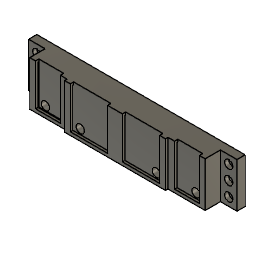
charging_plate (Autodesk Fusion 360 design; units mm, degrees)
part number: 2026-05-24-20-13-33-202
Autodesk Fusion 360 part; units mm, degrees
sketch "Sketch1" plane through (0, 0, 0) normal (0, 1, 0) x (1, 0, 0)
  line L0 (0, 0) -> (252, 0)
  line L1 (252, 0) -> (252, -54.2)
  line L2 (252, -54.2) -> (0, -54.2)
  line L3 (0, -54.2) -> (0, 0)
  dimension "d1" = 252
  dimension "d2" = 54.2
  constraint horizontal L0
  constraint vertical L1
  constraint horizontal L2
  constraint vertical L3
  constraint coincident L0.start L3.end
  measures "d1" distance of L0.start L0.end
  measures "d2" distance of L0.start L2.end
extrude "Extrude1" add sketch "Sketch1" along normal blind 10
sketch "Sketch2" plane through (0, 0, 0) normal (0, -1, 0) x (1, 0, 0)
  line L0 (252, 54.2) -> (0, 54.2)
  line L1 (0, 54.2) -> (0, 0)
  line L2 (0, 0) -> (252, 0)
  line L3 (252, 0) -> (252, 54.2)
  line L4 (20, 54.2) -> (232, 54.2)
  line L5 (232, 54.2) -> (232, 0)
  line L6 (232, 0) -> (20, 0)
  line L7 (20, 0) -> (20, 54.2)
  dimension "d5" = 20
  dimension "d6" = 20
  constraint horizontal L4
  constraint vertical L5
  constraint horizontal L6
  constraint vertical L7
  constraint coincident L2 L5.end
  constraint coincident L0 L4.start
  measures "d5" distance of L1.end L6.end
  measures "d6" distance of L2.end L5.end
extrude "Extrude2" add sketch "Sketch2" along normal blind 18.5 contours L0 L2 L4 L5 L6 L7
sketch "Sketch3" plane through (0, -18.5, 0) normal (0, -1, 0) x (1, 0, 0)
  line L0 (20, 0) -> (232, 0)
  line L1 (232, 0) -> (232, 54.2)
  line L2 (232, 54.2) -> (20, 54.2)
  line L3 (20, 54.2) -> (20, 0)
  line L4 (65, 54.2) -> (187, 54.2)
  line L5 (187, 54.2) -> (187, 0)
  line L6 (187, 0) -> (65, 0)
  line L7 (65, 0) -> (65, 54.2)
  dimension "d9" = 45
  dimension "d10" = 45
  constraint horizontal L4
  constraint vertical L5
  constraint horizontal L6
  constraint vertical L7
  constraint coincident L0 L5.end
  constraint coincident L2 L4.start
  measures "d9" distance of L0.start L6.end
  measures "d10" distance of L0.end L5.end
extrude "Extrude3" add sketch "Sketch3" along normal blind 3 contours L0 L2 L4 L5 L6 L7
sketch "Sketch4" plane through (0, -18.5, 0) normal (0, -1, 0) x (1, 0, 0)
  line L0 (65, 0) -> (65, 54.2)
  line L1 (65, 54.2) -> (20, 54.2)
  line L2 (20, 54.2) -> (20, 0)
  line L3 (20, 0) -> (65, 0)
  line L4 (27, 54.2) -> (57, 54.2)
  line L5 (57, 54.2) -> (57, 4)
  line L6 (57, 4) -> (27, 4)
  line L7 (27, 4) -> (27, 54.2)
  line L8 (195, 54.2) -> (225, 54.2)
  line L9 (225, 54.2) -> (225, 4)
  line L10 (225, 4) -> (195, 4)
  line L11 (195, 4) -> (195, 54.2)
  line L12 (232, 0) -> (252, 0)
  point P0 (232, 54.2)
  dimension "d13" = 7
  dimension "d14" = 30
  dimension "d15" = 4
  dimension "d16" = 7
  dimension "d17" = 30
  dimension "d18" = 4
  constraint horizontal L4
  constraint vertical L5
  constraint horizontal L6
  constraint vertical L7
  constraint coincident L1 L4.start
  constraint horizontal L8
  constraint vertical L9
  constraint horizontal L10
  constraint vertical L11
  measures "d13" distance of L1.end L4.start
  measures "d14" distance of L4.start L4.end
  measures "d15" distance of L3 L5.end
  measures "d16" distance of L8.end P0
  measures "d17" distance of L8.start L8.end
  measures "d18" distance of L9.end L12
extrude "Extrude4" cut sketch "Sketch4" against normal blind 4 contours L1 L4 L5 L6 L7 | L8 L9 L10 L11
sketch "Sketch5" plane through (0, 0, 4) normal (0, 0, 1) x (-1, 0, 0)
  line L0 (-27, 18.5) -> (-57, 18.5)
  line L1 (-57, 18.5) -> (-57, 14.5)
  line L2 (-57, 14.5) -> (-27, 14.5)
  line L3 (-27, 14.5) -> (-27, 18.5)
  line L4 (-24, 14.5285) -> (-59.9999, 14.5285)
  line L5 (-59.9999, 14.5285) -> (-59.9999, 15.5285)
  line L6 (-59.9999, 15.5285) -> (-24, 15.5285)
  line L7 (-24, 15.5285) -> (-24, 14.5285)
  line L8 (-192, 14.5) -> (-228, 14.5)
  line L9 (-228, 14.5) -> (-228, 15.5)
  line L10 (-228, 15.5) -> (-192, 15.5)
  line L11 (-192, 15.5) -> (-192, 14.5)
  line L12 (-195, 18.5) -> (-187, 18.5)
  point P0 (-195, 14.5)
  point P1 (-225, 14.5)
  dimension "d22" = 3
  dimension "d23" = 1
  dimension "d26" = 1
  dimension "d56" = 3
  dimension "d57" = 3
  dimension "d58" = 3
  dimension "d59" = 3
  constraint horizontal L4
  constraint vertical L5
  constraint horizontal L6
  constraint vertical L7
  constraint horizontal L8
  constraint vertical L9
  constraint horizontal L10
  constraint vertical L11
  measures "d22" distance of L1.end L4.end
  measures "d23" distance of L4.start L6.end
  measures "d26" distance of L8.end L9.end
  measures "d56" horizontal distance of L2.end L4.start
  measures "d57" distance of L8.start P0
  measures "d58" distance of L8.end P1
  measures "d59" distance of L10.end L12
extrude "Extrude5" cut sketch "Sketch5" along normal blind 47.2 and the other way blind 3 contours L3 L4 L6 L7 | L1 L3 L4 L6 | L1 L4 L5 L6 | L8 L9 L10 L11
sketch "Sketch6" plane through (0, -21.5, 0) normal (0, -1, 0) x (1, 0, 0)
  line L0 (65, 0) -> (187, 0)
  line L1 (187, 0) -> (187, 54.2)
  line L2 (187, 54.2) -> (65, 54.2)
  line L3 (65, 54.2) -> (65, 0)
  line L4 (72, 54.2) -> (117, 54.2)
  line L5 (117, 54.2) -> (117, 4)
  line L6 (117, 4) -> (72, 4)
  line L7 (72, 4) -> (72, 54.2)
  line L8 (180, 54.2) -> (135, 54.2)
  line L9 (135, 54.2) -> (135, 4)
  line L10 (135, 4) -> (180, 4)
  line L11 (180, 4) -> (180, 54.2)
  dimension "d31" = 7
  dimension "d32" = 45
  dimension "d33" = 4
  dimension "d34" = 7
  dimension "d35" = 45
  dimension "d36" = 4
  constraint horizontal L4
  constraint vertical L5
  constraint horizontal L6
  constraint vertical L7
  constraint coincident L2 L4.start
  constraint horizontal L8
  constraint vertical L9
  constraint horizontal L10
  constraint vertical L11
  constraint coincident L2 L8.start
  measures "d31" distance of L2.end L4.start
  measures "d32" distance of L4.start L4.end
  measures "d33" distance of L0 L6.end
  measures "d34" distance of L1.end L8.start
  measures "d35" distance of L8.start L8.end
  measures "d36" distance of L0 L9.end
extrude "Extrude6" cut sketch "Sketch6" against normal blind 4 contours L2 L4 L5 L6 L7 | L2 L8 L9 L10 L11
sketch "Sketch7" plane through (0, 0, 4) normal (0, 0, 1) x (-1, 0, 0)
  line L0 (-72, 21.5) -> (-117, 21.5)
  line L1 (-117, 17.5) -> (-72, 17.5)
  line L2 (-72, 17.5) -> (-72, 21.5)
  line L3 (-69, 17.5) -> (-120, 17.5)
  line L4 (-120, 17.5) -> (-120, 18.5)
  line L5 (-120, 18.5) -> (-69, 18.5)
  line L6 (-69, 18.5) -> (-69, 17.5)
  line L7 (-132, 17.5) -> (-183, 17.5)
  line L8 (-183, 17.5) -> (-183, 18.5)
  line L9 (-183, 18.5) -> (-132, 18.5)
  line L10 (-132, 18.5) -> (-132, 17.5)
  line L11 (-117, 21.5) -> (-117, 17.5)
  line L12 (-187, 21.5) -> (-180, 21.5)
  line L13 (-72, 21.5) -> (-65, 21.5)
  point P0 (-180, 17.5)
  point P1 (-135, 17.5)
  dimension "d41" = 1
  dimension "d45" = 1
  dimension "d60" = 3
  dimension "d61" = 3
  dimension "d62" = 3
  dimension "d63" = 3
  dimension "d64" = 3
  dimension "d65" = 3
  constraint horizontal L3
  constraint vertical L4
  constraint horizontal L5
  constraint vertical L6
  constraint horizontal L7
  constraint vertical L8
  constraint horizontal L9
  constraint vertical L10
  measures "d41" distance of L3.start L5.end
  measures "d45" distance of L7.end L8.end
  measures "d60" distance of L8.end L12
  measures "d61" distance of L7.end P0
  measures "d62" distance of L7.start P1
  measures "d63" distance of L5.end L13
  measures "d64" distance of L1.start L3.end
  measures "d65" distance of L1.end L3.start
extrude "Extrude7" cut sketch "Sketch7" along normal blind 47.2 and the other way blind 3 contours L2 L3 L5 L6 | L1 L2 L3 L5 L11 | L3 L4 L5 L11 | L7 L8 L9 L10
sketch "Sketch8" plane through (0, 10, 0) normal (0, 1, 0) x (-1, 0, 0)
  line L0 (0, 54.2) -> (-252, 54.2)
  line L1 (-252, 54.2) -> (-252, 0)
  line L2 (-252, 0) -> (0, 0)
  line L3 (0, 0) -> (0, 54.2)
  line L4 (-225, 44.2) -> (-27, 44.2)
  line L5 (-27, 44.2) -> (-27, 10)
  line L6 (-27, 10) -> (-225, 10)
  line L7 (-225, 10) -> (-225, 44.2)
  dimension "d50" = 27
  dimension "d51" = 27
  dimension "d52" = 10
  dimension "d53" = 10
  constraint horizontal L4
  constraint vertical L5
  constraint horizontal L6
  constraint vertical L7
  measures "d50" distance of L1 L7
  measures "d51" distance of L3 L5
  measures "d52" distance of L0 L4
  measures "d53" distance of L2 L6
extrude "Extrude8" cut sketch "Sketch8" against normal blind 20 contours L4 L5 L6 L7
sketch "Sketch9" plane through (0, -10, 0) normal (0, 1, 0) x (-1, 0, 0)
  line L0 (-225, 10) -> (-27, 10)
  line L1 (-27, 10) -> (-27, 44.2)
  line L2 (-27, 44.2) -> (-225, 44.2)
  line L3 (-225, 44.2) -> (-225, 10)
  circle A0 centre (-217, 9.2) radius 5
  circle A1 centre (-172, 9.2) radius 5
  circle A2 centre (-80, 9.2) radius 5
  circle A3 centre (-35, 9.2) radius 5
  line L4 (-252, 54.2) -> (-252, 0)
  line L5 (0, 54.2) -> (0, 0)
  line L6 (0, 54.2) -> (-252, 54.2)
  dimension "d66" = 10
  dimension "d67" = 80
  dimension "d68" = 35
  dimension "d69" = 35
  dimension "d70" = 80
  dimension "d71" = 45
  dimension "d72" = 45
  dimension "d73" = 45
  dimension "d74" = 45
  constraint equal A0 A1
  constraint equal A0 A2
  constraint equal A0 A3
  measures "d66" diameter of A0
  measures "d67" distance of A1.centre L4
  measures "d68" distance of A0.centre L4
  measures "d69" distance of A3.centre L5
  measures "d70" distance of A2.centre L5
  measures "d71" distance of A0.centre L6
  measures "d72" distance of A1.centre L6
  measures "d73" distance of A2.centre L6
  measures "d74" distance of A3.centre L6
extrude "Extrude9" cut sketch "Sketch9" along normal up to surface (-7.5 mm away) and the other way up to surface (-20 mm away) contours L0 A0 | L0 A0 | L0 A1 | L0 A1 | L0 A3 | L0 A3 | L0 A2 | L0 A2
sketch "Sketch10" plane through (0, 0, 0) normal (0, -1, 0) x (1, 0, 0)
  line L0 (20, 0) -> (20, 54.2)
  line L1 (20, 54.2) -> (0, 54.2)
  line L2 (0, 54.2) -> (0, 0)
  line L3 (0, 0) -> (20, 0)
  circle A0 centre (10, 27.1) radius 5
  circle A1 centre (10, 10) radius 5
  circle A2 centre (10, 44.2) radius 5
  circle A3 centre (242, 27.1) radius 5
  circle A4 centre (242, 44.2) radius 5
  circle A5 centre (242, 10) radius 5
  line L4 (252, 0) -> (252, 54.2)
  line L5 (232, 0) -> (252, 0)
  line L6 (252, 54.2) -> (232, 54.2)
  dimension "d77" = 10
  dimension "d78" = 10
  dimension "d79" = 27.1
  dimension "d80" = 10
  dimension "d81" = 10
  dimension "d82" = 10
  dimension "d83" = 10
  dimension "d84" = 10
  dimension "d85" = 10
  dimension "d86" = 10
  dimension "d87" = 27.1
  dimension "d88" = 10
  dimension "d89" = 10
  constraint equal A0 A2
  constraint equal A0 A1
  constraint equal A0 A5
  constraint equal A0 A4
  constraint equal A0 A3
  measures "d77" diameter of A0
  measures "d78" distance of L2 A0.centre
  measures "d79" distance of L3 A0.centre
  measures "d80" distance of L2 A2.centre
  measures "d81" distance of L2 A1.centre
  measures "d82" distance of L1 A2.centre
  measures "d83" distance of L3 A1.centre
  measures "d84" distance of A3.centre L4
  measures "d85" distance of A4.centre L4
  measures "d86" distance of A5.centre L4
  measures "d87" distance of A3.centre L5
  measures "d88" distance of A4.centre L6
  measures "d89" distance of A5.centre L5
extrude "Extrude10" cut sketch "Sketch10" against normal blind 5 contours A0 | A1 | A2 | A3 | A4 | A5
sketch "Sketch11" plane through (0, 5, 0) normal (0, -1, 0) x (1, 0, 0)
  circle A0 centre (10, 44.2) radius 5
  circle A1 centre (10, 44.2) radius 1.65
  circle A2 centre (10, 27) radius 1.65
  circle A3 centre (10, 10) radius 1.65
  circle A4 centre (242.104, 44.4888) radius 1.65
  circle A5 centre (242, 27) radius 1.65
  circle A6 centre (242, 10) radius 1.65
  dimension "d92" = 3.3
  dimension "d93" = 3.3
  dimension "d94" = 3.3
  dimension "d95" = 3.3
  dimension "d96" = 3.3
  dimension "d97" = 3.3
  constraint concentric A0 A1
  measures "d92" diameter of A1
  measures "d93" diameter of A2
  measures "d94" diameter of A3
  measures "d95" diameter of A4
  measures "d96" diameter of A5
  measures "d97" diameter of A6
extrude "Extrude11" cut sketch "Sketch11" against normal blind 5 contours A1 | A2 | A3 | A4 | A5 | A6
